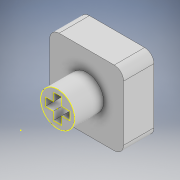
# Autodesk Inventor part: IPC RCL key
Saved by Autodesk Inventor 2022 (Build 260153000, 153)
## iProperties
Created: 2021-12-31
Part Number: IPC RCL key
Material: Generic
Document SubType Name: Modeling
Designer: solor
Density: 1 g/cm^3
Appearance: Default
Author: solor
Autodesk Inventor part; units mm, degrees
ref_plane "YZ Plane" through (0, 0, 0) normal (1, 0, 0) x (0, 1, 0)
ref_plane "XZ Plane" through (0, 0, 0) normal (0, 1, 0) x (-1, 0, 0)
sketch "Sketch1" plane through (0, 0, 0) normal (0, 0, 1) x (1, 0, 0)
  line L0 (14.6962, 12.74) -> (14.6962, 0) construction
  line L1 (10.61, 12.2) -> (1.53, 12.2)
  arc A0 (1.53, 12.2) -> (0, 10.67) centre (1.53, 10.67) ccw
  line L2 (0, 10.67) -> (0, 1.53)
  arc A1 (0, 1.53) -> (1.53, 0) centre (1.53, 1.53) ccw
  line L3 (1.53, 0) -> (10.61, 0)
  arc A2 (10.61, 0) -> (12.14, 1.53) centre (10.61, 1.53) ccw
  arc A3 (12.14, 10.67) -> (10.61, 12.2) centre (10.61, 10.67) ccw
  line L4 (12.14, 10.67) -> (12.14, 1.53)
  point P0 (0, 0)
  point P1 (0, 0)
  dimension "d10" = 12.74
  constraints: 10 end point, 8 point on circle, 4 centre point, 2 vertical, 1 point on line
  measures "d10" distance of L0.start L0.end
ref_plane "Work Plane1" through (0, 0, 5) normal (0, 0, 1) x (1, 0, 0)
sketch "Sketch2" plane through (0, 0, 5) normal (0, 0, 1) x (1, 0, 0)
  line L0 (10.88, 12.74) -> (1.8, 12.74) projected
  line L1 (10.88, 12.74) -> (1.8, 12.74) projected
  arc A0 (1.8, 12.74) -> (0, 10.94) centre (1.8, 10.94) ccw projected
  line L2 (0, 10.94) -> (0, 1.8) projected
  arc A1 (0, 1.8) -> (1.8, 0) centre (1.8, 1.8) ccw projected
  line L3 (1.8, 0) -> (10.88, 0) projected
  arc A2 (10.88, 0) -> (12.68, 1.8) centre (10.88, 1.8) ccw projected
  line L4 (12.68, 1.8) -> (12.68, 10.94) projected
  arc A3 (12.68, 10.94) -> (10.88, 12.74) centre (10.88, 10.94) ccw projected
  circle A4 centre (6.34, 6.37) radius 2.8
  line L5 (5.665, 8.395) -> (7.015, 8.395)
  line L6 (7.015, 4.345) -> (5.665, 4.345)
  line L7 (5.665, 4.345) -> (7.015, 8.395) construction
  line L8 (5.665, 8.395) -> (7.015, 4.345) construction
  line L9 (8.365, 5.695) -> (8.365, 7.045)
  line L10 (4.315, 7.045) -> (4.315, 5.695)
  line L11 (4.315, 5.695) -> (8.365, 7.045) construction
  line L12 (8.365, 5.695) -> (4.315, 7.045) construction
  line L13 (4.315, 5.695) -> (5.665, 5.695)
  line L14 (7.015, 5.695) -> (8.365, 5.695)
  line L15 (5.665, 4.345) -> (5.665, 5.695)
  line L16 (5.665, 7.045) -> (5.665, 8.395)
  line L17 (8.365, 7.045) -> (7.015, 7.045)
  line L18 (5.665, 7.045) -> (4.315, 7.045)
  line L19 (7.015, 8.395) -> (7.015, 7.045)
  line L20 (7.015, 5.695) -> (7.015, 4.345)
  point P0 (0, 0)
  dimension "d3" = 5.6
  dimension "d4" = 4.05
  dimension "d5" = 1.35
  dimension "d6" = 4.05
  dimension "d7" = 1.35
  constraints: 32 end point, 10 parallel, 8 perpendicular, 4 midpoint, 2 vertical, 1 centre point
  measures "d3" diameter of A4
  measures "d4" distance of L6.end L5.start
  measures "d5" distance of L5.start L5.end
  measures "d6" distance of L10.end L9.start
  measures "d7" distance of L9.end L9.start
extrude "Extrusion3" add sketch "Sketch1" along normal blind 5
sketch "Sketch3" plane through (0, 0, 5) normal (0, 0, 1) x (1, 0, 0)
  line L0 (10.61, 12.47) -> (1.53, 12.47)
  line L1 (10.61, 12.47) -> (1.53, 12.47)
  arc A0 (1.53, 12.47) -> (-0.27, 10.67) centre (1.53, 10.67) ccw
  line L2 (-0.27, 10.67) -> (-0.27, 1.53)
  arc A1 (-0.27, 1.53) -> (1.53, -0.27) centre (1.53, 1.53) ccw
  line L3 (1.53, -0.27) -> (10.61, -0.27)
  arc A2 (10.61, -0.27) -> (12.41, 1.53) centre (10.61, 1.53) ccw
  line L4 (12.41, 1.53) -> (12.41, 10.67)
  arc A3 (12.41, 10.67) -> (10.61, 12.47) centre (10.61, 10.67) ccw
  circle A4 centre (6.07, 6.1) radius 2.8
  line L5 (5.395, 8.125) -> (6.745, 8.125)
  line L6 (6.745, 4.075) -> (5.395, 4.075)
  line L7 (5.395, 4.075) -> (6.745, 8.125) construction
  line L8 (5.395, 8.125) -> (6.745, 4.075) construction
  line L9 (8.095, 5.425) -> (8.095, 6.775)
  line L10 (4.045, 6.775) -> (4.045, 5.425)
  line L11 (4.045, 5.425) -> (8.095, 6.775) construction
  line L12 (8.095, 5.425) -> (4.045, 6.775) construction
  line L13 (4.045, 5.425) -> (5.395, 5.425)
  line L14 (6.745, 5.425) -> (8.095, 5.425)
  line L15 (5.395, 4.075) -> (5.395, 5.425)
  line L16 (5.395, 6.775) -> (5.395, 8.125)
  line L17 (8.095, 6.775) -> (6.745, 6.775)
  line L18 (5.395, 6.775) -> (4.045, 6.775)
  line L19 (6.745, 8.125) -> (6.745, 6.775)
  line L20 (6.745, 5.425) -> (6.745, 4.075)
  line L21 (10.61, 12.2) -> (1.53, 12.2) projected
  line L22 (0, 10.67) -> (0, 1.53) projected
  point P0 (0, 0)
  point P1 (-0.27, -0.27)
  point P2 (6.07, 12.2)
  point P3 (0, 6.1)
  point P4 (6.07, 6.1)
  dimension "d14" = 5.6
  dimension "d15" = 4.05
  dimension "d16" = 1.35
  dimension "d17" = 4.05
  dimension "d18" = 1.35
  constraints: 42 end point, 10 parallel, 8 perpendicular, 8 point on circle, 6 midpoint, 5 centre point, 2 vertical
  measures "d14" diameter of A4
  measures "d15" distance of L6.end L5.start
  measures "d16" distance of L5.start L5.end
  measures "d17" distance of L10.end L9.start
  measures "d18" distance of L9.end L9.start
extrude "Extrusion4" add sketch "Sketch3" along normal blind 4.8 contours A4
sketch "Sketch4" plane through (0, 0, 0) normal (0, 0, -1) x (-1, 0, 0)
  line L0 (-13.9436, 0) -> (-13.9436, 2.266)
  line L1 (-15.5559, 0) -> (-15.5559, 6.84)
  line L2 (-1.53, 0) -> (-10.61, 0) projected
  line L3 (-10.1927, 7.6843) -> (-1.9473, 7.6843) construction
  line L4 (-1.9473, 7.6843) -> (-1.9473, 4.5157) construction
  line L5 (-1.9473, 4.5157) -> (-10.1927, 4.5157) construction
  line L6 (-10.1927, 4.5157) -> (-10.1927, 7.6843) construction
  line L7 (-7.0587, 4.575) -> (-7.9905, 4.575)
  line L8 (-7.9905, 4.575) -> (-8.8382, 5.6947)
  line L9 (-8.8382, 5.6947) -> (-9.1151, 5.6947)
  line L10 (-9.1151, 5.6947) -> (-9.1151, 4.575)
  line L11 (-9.1151, 4.575) -> (-9.8763, 4.575)
  line L12 (-9.8763, 4.575) -> (-9.8763, 7.625)
  line L13 (-9.8763, 7.625) -> (-8.6504, 7.625)
  spline S0 degree 2 poles (-8.6504, 7.625) (-8.3958, 7.625) (-8.0201, 7.5607) (-7.8595, 7.4619) knots 0 0 0 1 2 2 2
  spline S1 degree 2 poles (-7.8595, 7.4619) (-7.6963, 7.3581) (-7.5035, 7.0343) (-7.5035, 6.7871) knots 0 0 0 1 2 2 2
  spline S2 degree 2 poles (-7.5035, 6.7871) (-7.5035, 6.4386) (-7.8199, 6.0011) (-8.0844, 5.8726) knots 0 0 0 1 2 2 2
  line L14 (-8.0844, 5.8726) -> (-7.0587, 4.575)
  spline S3 degree 2 poles (-8.2895, 6.6907) (-8.2895, 6.8069) (-8.3785, 6.9725) (-8.4798, 7.017) knots 0 0 0 1 2 2 2
  spline S4 degree 2 poles (-8.4798, 7.017) (-8.5515, 7.0466) (-8.727, 7.0639) (-8.858, 7.0639) knots 0 0 0 1 2 2 2
  line L15 (-8.858, 7.0639) -> (-9.1151, 7.0639)
  line L16 (-9.1151, 7.0639) -> (-9.1151, 6.2434)
  line L17 (-9.1151, 6.2434) -> (-8.8951, 6.2434)
  spline S5 degree 2 poles (-8.8951, 6.2434) (-8.7369, 6.2434) (-8.512, 6.2829) (-8.4354, 6.3447) knots 0 0 0 1 2 2 2
  spline S6 degree 2 poles (-8.4354, 6.3447) (-8.3612, 6.404) (-8.2895, 6.5622) (-8.2895, 6.6907) knots 0 0 0 1 2 2 2
  spline S7 degree 2 poles (-5.5164, 4.5157) (-6.2035, 4.5157) (-7.0092, 5.3462) (-7.0092, 6.0975) knots 0 0 0 1 2 2 2
  spline S8 degree 2 poles (-7.0092, 6.0975) (-7.0092, 6.8217) (-6.201, 7.6843) (-5.5139, 7.6843) knots 0 0 0 1 2 2 2
  spline S9 degree 2 poles (-5.5139, 7.6843) (-5.3335, 7.6843) (-5.0418, 7.6423) (-4.9083, 7.6077) knots 0 0 0 1 2 2 2
  spline S10 degree 2 poles (-4.9083, 7.6077) (-4.8045, 7.5756) (-4.5598, 7.4693) (-4.4832, 7.4297) knots 0 0 0 1 2 2 2
  line L18 (-4.4832, 7.4297) -> (-4.4832, 6.7031)
  line L19 (-4.4832, 6.7031) -> (-4.5598, 6.7031)
  spline S11 degree 2 poles (-4.5598, 6.7031) (-4.6167, 6.7525) (-4.7847, 6.8909) (-4.891, 6.9552) knots 0 0 0 1 2 2 2
  spline S12 degree 2 poles (-4.891, 6.9552) (-4.9973, 7.0219) (-5.2519, 7.1134) (-5.3928, 7.1134) knots 0 0 0 1 2 2 2
  spline S13 degree 2 poles (-5.3928, 7.1134) (-5.5584, 7.1134) (-5.8327, 7.0096) (-5.9588, 6.8786) knots 0 0 0 1 2 2 2
  spline S14 degree 2 poles (-5.9588, 6.8786) (-6.0725, 6.7624) (-6.2183, 6.3645) (-6.2183, 6.0951) knots 0 0 0 1 2 2 2
  spline S15 degree 2 poles (-6.2183, 6.0951) (-6.2183, 5.8108) (-6.0675, 5.4228) (-5.9439, 5.3041) knots 0 0 0 1 2 2 2
  spline S16 degree 2 poles (-5.9439, 5.3041) (-5.8253, 5.188) (-5.5337, 5.0866) (-5.3878, 5.0866) knots 0 0 0 1 2 2 2
  spline S17 degree 2 poles (-5.3878, 5.0866) (-5.2371, 5.0866) (-4.9627, 5.188) (-4.8688, 5.2498) knots 0 0 0 1 2 2 2
  spline S18 degree 2 poles (-4.8688, 5.2498) (-4.765, 5.3115) (-4.6093, 5.4425) (-4.5524, 5.4944) knots 0 0 0 1 2 2 2
  line L20 (-4.5524, 5.4944) -> (-4.4832, 5.4944)
  line L21 (-4.4832, 5.4944) -> (-4.4832, 4.7777)
  spline S19 degree 2 poles (-4.4832, 4.7777) (-4.5672, 4.7381) (-4.7872, 4.6393) (-4.9059, 4.6047) knots 0 0 0 1 2 2 2
  spline S20 degree 2 poles (-4.9059, 4.6047) (-5.0492, 4.5602) (-5.2988, 4.5157) (-5.5164, 4.5157) knots 0 0 0 1 2 2 2
  line L22 (-1.9967, 4.575) -> (-4.0309, 4.575)
  line L23 (-4.0309, 4.575) -> (-4.0309, 7.625)
  line L24 (-4.0309, 7.625) -> (-3.2647, 7.625)
  line L25 (-3.2647, 7.625) -> (-3.2647, 5.1558)
  line L26 (-3.2647, 5.1558) -> (-1.9967, 5.1558)
  line L27 (-1.9967, 5.1558) -> (-1.9967, 4.575)
  point P0 (0, 0)
  point P1 (-6.07, 0)
  point P2 (-6.07, 2.266)
  point P3 (-6.07, 6.1)
  point P4 (-6.07, 6.84)
  point P5 (-6.07, 4.5157)
  point P6 (-1.9473, 6.1)
  point P7 (-6.07, 6.1)
  dimension "d21" = 2.266
  dimension "d22" = 6.84
  constraints: 4 end point, 3 midpoint, 2 vertical, 2 other
  measures "d21" distance of L0.start L0.end
  measures "d22" distance of L1.start L1.end
extrude "Extrusion5" add sketch "Sketch4" along normal blind 0.9
sketch "Sketch5" plane through (6.07, 6.1, 9.8) normal (0, 0, 1) x (1, 0, 0)
  circle A0 centre (0, 0) radius 2.8 projected
  line L0 (-0.675, 0.675) -> (-0.675, 2.025) projected
  line L1 (-0.675, 2.025) -> (0.675, 2.025) projected
  line L2 (0.675, 2.025) -> (0.675, 0.675) projected
  line L3 (0.675, 0.675) -> (2.025, 0.675) projected
  line L4 (2.025, 0.675) -> (2.025, -0.675) projected
  line L5 (2.025, -0.675) -> (0.675, -0.675) projected
  line L6 (0.675, -0.675) -> (0.675, -2.025) projected
  line L7 (0.675, -2.025) -> (-0.675, -2.025) projected
  line L8 (-0.675, -2.025) -> (-0.675, -0.675) projected
  line L9 (-0.675, -0.675) -> (-2.025, -0.675) projected
  line L10 (-2.025, -0.675) -> (-2.025, 0.675) projected
  line L11 (-2.025, 0.675) -> (-0.675, 0.675) projected
  point P0 (-6.07, -6.1)
body "Solid2"
